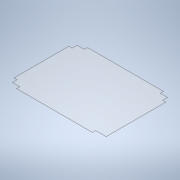
# Autodesk Inventor part: Cut Lexan DriveTrain
Saved by Autodesk Inventor 2020 (Build 240168000, 168)
## iProperties
Created: 2020-01-14
Part Number: Cut Lexan DriveTrain
Material: Polycarbonate, Clear
Document SubType Name: Modeling
Designer: aidan
Density: 1.2 g/cm^3
Appearance: Polycarbonate - Clear
Author: aidan
Autodesk Inventor part; units mm, degrees
ref_plane "YZ Plane" through (0, 0, 0) normal (1, 0, 0) x (0, 1, 0)
sketch "Sketch1" plane through (0, 0, 0) normal (0, 1, 0) x (-1, 0, 0)
  line L0 (374.9202, 295.3426) -> (-387.0798, 295.3426)
  line L1 (-387.0798, 295.3426) -> (-387.0798, -263.4574)
  line L2 (-387.0798, -263.4574) -> (374.9202, -263.4574)
  line L3 (374.9202, -263.4574) -> (374.9202, 295.3426)
  point P0 (0, 0)
  dimension "d0" = 558.8
  dimension "d1" = 762
  constraints: 8 end point, 2 parallel, 1 horizontal, 1 perpendicular
  measures "d0" distance of L2.end L0.start
  measures "d1" distance of L1.end L2.end
extrude "Extrusion1" add sketch "Sketch1" along normal blind 2.9972
sketch "Sketch2" plane through (0, 2.9972, 0) normal (0, 1, 0) x (1, 0, 0)
  line L0 (-374.9202, -231.8426) -> (-374.9202, -295.3426)
  line L1 (-374.9202, -295.3426) -> (-292.3702, -295.3426)
  line L2 (-292.3702, -295.3426) -> (-292.3702, -269.9426)
  line L3 (-292.3702, -269.9426) -> (-349.5202, -269.9426)
  line L4 (-349.5202, -269.9426) -> (-349.5202, -231.8426)
  line L5 (-349.5202, -231.8426) -> (-374.9202, -231.8426)
  line L6 (-374.9202, 263.4574) -> (-374.9202, -295.3426) projected
  line L7 (-374.9202, -295.3426) -> (387.0798, -295.3426) projected
  point P0 (0, 0)
  dimension "d4" = 63.5
  dimension "d5" = 82.55
  dimension "d6" = 25.4
  dimension "d7" = 25.4
  constraints: 12 end point, 2 collinear, 2 perpendicular, 1 horizontal, 1 parallel, 1 vertical
  measures "d4" distance of L0.start L0.end
  measures "d5" distance of L0.end L1.end
  measures "d6" distance of L1.end L2.end
  measures "d7" distance of L4.end L0.start
extrude "Extrusion2" cut sketch "Sketch2" against normal blind 2.9972
ref_plane "Work Plane3" through (-292.3702, 0, 15.9426) normal (0, 0, 1) x (1, 0, 0)
mirror "Mirror1" about plane through (-292.3702, 0, 15.9426) normal (0, 0, 1) of "Extrusion2"
ref_plane "Work Plane4" through (6.0798, 0, -199.9574) normal (-1, 0, 0) x (0, 0, 1)
mirror "Mirror2" about plane through (6.0798, 0, -199.9574) normal (-1, 0, 0) of "Extrusion2", "Mirror1"
sketch "Sketch3" plane through (0, 2.9972, 0) normal (0, 1, 0) x (1, 0, 0)
  line L0 (387.0798, -231.8426) -> (387.0798, 199.9574) projected
  line L1 (304.5298, -269.9426) -> (361.6798, -269.9426) projected
  line L2 (387.0798, -231.8426) -> (361.6798, -231.8426)
  line L3 (361.6798, -231.8426) -> (361.6798, -269.9426)
  line L4 (361.6798, -269.9426) -> (387.0798, -269.9426)
  line L5 (387.0798, -269.9426) -> (387.0798, -231.8426)
  point P0 (0, 0)
  constraints: 8 end point, 2 parallel, 1 horizontal, 1 perpendicular
extrude "Extrusion3" add sketch "Sketch3" against normal blind 2.9972
body "Solid1"
